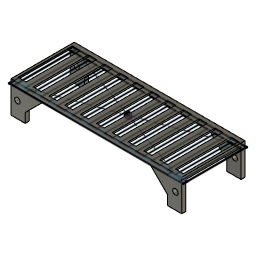
Rear Vent Grill (2mm Smaller) (Autodesk Fusion 360 design; units mm, degrees)
Autodesk Fusion 360 part; units mm, degrees
sketch "Sketch1" plane through (0, 0, 0) normal (0, 0, 1) x (1, 0, 0)
  line L0 (55, -20) -> (-55, -20)
  line L1 (-55, -20) -> (-55, 20)
  line L2 (-55, 20) -> (55, 20)
  line L3 (55, 20) -> (55, -20)
  line L4 (55, -20) -> (-55, 20) construction
  line L5 (-55, -20) -> (55, 20) construction
  line L6 (-55, 20) -> (-52.5, 20)
  line L7 (-52.5, 20) -> (-52.5, -20)
  line L8 (-52.5, -20) -> (-55, -20)
  line L9 (-55, -20) -> (-55, 20)
  line L10 (55, 20) -> (52.5, 20)
  line L11 (52.5, 20) -> (52.5, -20)
  line L12 (52.5, -20) -> (55, -20)
  line L13 (55, -20) -> (55, 20)
  line L14 (-55, 20) -> (55, 20)
  line L15 (55, 20) -> (55, 17.5)
  line L16 (55, 17.5) -> (-55, 17.5)
  line L17 (-55, 17.5) -> (-55, 20)
  line L18 (-55, -20) -> (55, -20)
  line L19 (55, -20) -> (55, -17.5)
  line L20 (55, -17.5) -> (-55, -17.5)
  line L21 (-55, -17.5) -> (-55, -20)
  line L22 (-52.5, 17.5) -> (-47.5, 17.5)
  line L23 (-47.5, 17.5) -> (-47.5, -17.5)
  line L24 (-47.5, -17.5) -> (-52.5, -17.5)
  line L25 (-52.5, -17.5) -> (-52.5, 17.5)
  line L26 (-42.5, -17.5) -> (-42.5, 17.5)
  line L27 (-42.5, 17.5) -> (-37.5, 17.5)
  line L28 (-37.5, 17.5) -> (-37.5, -17.5)
  line L29 (-37.5, -17.5) -> (-42.5, -17.5)
  line L30 (-32.5, -17.5) -> (-32.5, 17.5)
  line L31 (-32.5, 17.5) -> (-27.5, 17.5)
  line L32 (-27.5, 17.5) -> (-27.5, -17.5)
  line L33 (-27.5, -17.5) -> (-32.5, -17.5)
  line L34 (-22.5, -17.5) -> (-22.5, 17.5)
  line L35 (-22.5, 17.5) -> (-17.5, 17.5)
  line L36 (-17.5, 17.5) -> (-17.5, -17.5)
  line L37 (-17.5, -17.5) -> (-22.5, -17.5)
  line L38 (-12.5, -17.5) -> (-12.5, 17.5)
  line L39 (-12.5, 17.5) -> (-7.5, 17.5)
  line L40 (-7.5, 17.5) -> (-7.5, -17.5)
  line L41 (-7.5, -17.5) -> (-12.5, -17.5)
  line L42 (-2.5, -17.5) -> (-2.5, 17.5)
  line L43 (-2.5, 17.5) -> (2.5, 17.5)
  line L44 (2.5, 17.5) -> (2.5, -17.5)
  line L45 (2.5, -17.5) -> (-2.5, -17.5)
  line L46 (7.5, -17.5) -> (7.5, 17.5)
  line L47 (7.5, 17.5) -> (12.5, 17.5)
  line L48 (12.5, 17.5) -> (12.5, -17.5)
  line L49 (12.5, -17.5) -> (7.5, -17.5)
  line L50 (17.5, -17.5) -> (17.5, 17.5)
  line L51 (17.5, 17.5) -> (22.5, 17.5)
  line L52 (22.5, 17.5) -> (22.5, -17.5)
  line L53 (22.5, -17.5) -> (17.5, -17.5)
  line L54 (27.5, -17.5) -> (27.5, 17.5)
  line L55 (27.5, 17.5) -> (32.5, 17.5)
  line L56 (32.5, 17.5) -> (32.5, -17.5)
  line L57 (32.5, -17.5) -> (27.5, -17.5)
  line L58 (37.5, -17.5) -> (37.5, 17.5)
  line L59 (37.5, 17.5) -> (42.5, 17.5)
  line L60 (42.5, 17.5) -> (42.5, -17.5)
  line L61 (42.5, -17.5) -> (37.5, -17.5)
  line L62 (47.5, -17.5) -> (47.5, 17.5)
  line L63 (47.5, 17.5) -> (52.5, 17.5)
  line L64 (52.5, 17.5) -> (52.5, -17.5)
  line L65 (52.5, -17.5) -> (47.5, -17.5)
  line L66 (-55, -20) -> (-45, -20)
  line L67 (-45, -20) -> (-45, -17)
  line L68 (-45, -17) -> (-55, -17)
  line L69 (-55, -17) -> (-55, -20)
  line L70 (-55, 20) -> (-45, 20)
  line L71 (-45, 20) -> (-45, 17)
  line L72 (-45, 17) -> (-55, 17)
  line L73 (-55, 17) -> (-55, 20)
  line L74 (55, -20) -> (45, -20)
  line L75 (45, -20) -> (45, -17)
  line L76 (45, -17) -> (55, -17)
  line L77 (55, -17) -> (55, -20)
  line L78 (55, 20) -> (45, 20)
  line L79 (45, 20) -> (45, 17)
  line L80 (45, 17) -> (55, 17)
  line L81 (55, 17) -> (55, 20)
  dimension "d1" = 40
  dimension "d2" = 110
  dimension "d3" = 2.5
  dimension "d4" = 2.5
  dimension "d5" = 2.5
  dimension "d6" = 2.5
  dimension "d7" = 5
  dimension "d10" = 100
  dimension "d11" = 0
  dimension "d14" = 3
  dimension "d15" = 10
  dimension "d16" = 10
  dimension "d17" = 3
  dimension "d18" = 10
  dimension "d19" = 3
  dimension "d20" = 3
  dimension "d21" = 10
  constraint perpendicular L0 L1
  constraint parallel L0 L2
  constraint parallel L1 L3
  constraint horizontal L0
  constraint coincident L4 origin
  constraint coincident L5 origin
  constraint horizontal L6
  constraint vertical L7
  constraint horizontal L8
  constraint vertical L9
  constraint horizontal L10
  constraint vertical L11
  constraint horizontal L12
  constraint vertical L13
  constraint horizontal L14
  constraint vertical L15
  constraint horizontal L16
  constraint vertical L17
  constraint horizontal L18
  constraint vertical L19
  constraint horizontal L20
  constraint vertical L21
  constraint horizontal L22
  constraint vertical L23
  constraint horizontal L24
  constraint vertical L25
  constraint coincident L7 L22.start
  constraint coincident L16 L22.start
  constraint horizontal L66
  constraint vertical L67
  constraint horizontal L68
  constraint vertical L69
  constraint horizontal L70
  constraint vertical L71
  constraint horizontal L72
  constraint vertical L73
  constraint horizontal L74
  constraint vertical L75
  constraint horizontal L76
  constraint vertical L77
  constraint horizontal L78
  constraint vertical L79
  constraint horizontal L80
  constraint vertical L81
  measures "d1" distance of L0.end L1.end
  measures "d2" distance of L1.end L2.end
  measures "d3" distance of L1.end L6.end
  measures "d4" distance of L2.end L10.end
  measures "d5" distance of L1.end L16.end
  measures "d6" distance of L0.end L20.end
  measures "d7" distance of L22.start L22.end
  measures "d14" distance of L0.end L68.end
  measures "d15" distance of L0.end L66.end
  measures "d16" distance of L1.end L70.end
  measures "d17" distance of L1.end L72.end
  measures "d18" distance of L0.start L74.end
  measures "d19" distance of L0.start L76.end
  measures "d20" distance of L2.end L80.end
  measures "d21" distance of L2.end L78.end
extrude "Extrude1" add sketch "Sketch1" along normal blind 3 contours L0 L3 L11 L12 L13 L18 L19 L20 L74 L77 | L0 L11 L18 L20 L65 L74 L75 | L3 L11 L13 L20 L64 L76 L77 | L0 L18 L20 L29 L33 L37 L41 L45 L49 L53 L57 L61 L67 L75 | L3 L11 L13 L64 L76 L80 | L0 L7 L18 L20 L24 L66 L67 | L20 L62 L75 L76 | L16 L20 L60 L62 L75 L76 L79 L80 | L3 L11 L13 L16 L64 L80 L81 | L0 L1 L7 L8 L9 L18 L20 L21 L66 L69 | L16 L20 L23 L26 L67 L68 L71 L72 | L2 L3 L10 L11 L13 L14 L15 L16 L78 L81 | L1 L7 L9 L20 L25 L68 L69 | L7 L20 L23 L24 L25 L68 | L16 L20 L56 L58 | L2 L14 L16 L27 L31 L35 L39 L43 L47 L51 L55 L59 L71 L79 | L2 L11 L14 L16 L63 L78 L79 | L16 L62 L79 L80 | L1 L7 L9 L25 L68 L72 | L16 L20 L28 L30 | L1 L7 L9 L16 L25 L72 L73 | L7 L16 L22 L23 L25 L72 | L2 L7 L14 L16 L22 L70 L71 | L16 L20 L52 L54 | L1 L2 L6 L7 L9 L14 L16 L17 L70 L73 | L16 L20 L32 L34 | L16 L20 L48 L50 | L16 L20 L36 L38 | L16 L20 L44 L46 | L16 L20 L40 L42
extrude "Extrude2" add sketch "Sketch1" against normal blind 17 contours L0 L3 L11 L12 L13 L18 L19 L20 L74 L77 | L0 L11 L18 L20 L65 L74 L75 | L0 L7 L18 L20 L24 L66 L67 | L0 L1 L7 L8 L9 L18 L20 L21 L66 L69 | L2 L3 L10 L11 L13 L14 L15 L16 L78 L81 | L2 L11 L14 L16 L63 L78 L79 | L2 L7 L14 L16 L22 L70 L71 | L1 L2 L6 L7 L9 L14 L16 L17 L70 L73
sketch "Sketch2" plane through (0, -20, 0) normal (0, -1, 0) x (1, 0, 0)
  line L0 (-45, 0) -> (45, 0)
  line L1 (45, 0) -> (45, -17)
  line L2 (45, -17) -> (55, -17)
  line L3 (55, -17) -> (55, 3)
  line L4 (55, 3) -> (-55, 3)
  line L5 (-55, 3) -> (-55, -17)
  line L6 (-55, -17) -> (-45, -17)
  line L7 (-45, -17) -> (-45, 0)
  circle A0 centre (-50, -7) radius 1.75
  circle A1 centre (50, -7) radius 1.75
  dimension "d24" = 3.5
  dimension "d25" = 3.5
  dimension "d28" = 10
  dimension "d29" = 10
  dimension "d30" = 5
  dimension "d31" = 5
  measures "d24" diameter of A0
  measures "d25" diameter of A1
  measures "d28" distance of L4 A1.centre
  measures "d29" distance of L4 A0.centre
  measures "d30" distance of L5 A0.centre
  measures "d31" distance of L3 A1.centre
extrude "Extrude3" cut sketch "Sketch2" against normal up to surface (40 mm away) contours A0 | A1
extrude "Extrude4" add 1 faces at (-45.8333, 17, 1) along direction (0, 1, 0) blind 0.5
extrude "Extrude5" add 1 faces at (-45.8333, -17, 1) along direction (0, -1, 0) blind 0.5
chamfer "Chamfer1" distance 2 angle 45 19 edges at (47.5, 0, 0) (42.5, 0, 0) (37.5, 0, 0) (32.5, 0, 0) (22.5, 0, 0) (27.5, 0, 0) (17.5, 0, 0) (12.5, 0, 0) (7.5, 0, 0) (2.5, 0, 0) (-2.5, 0, 0) (-7.5, 0, 0) (-12.5, 0, 0) (-17.5, 0, 0) (-22.5, 0, 0) (-27.5, 0, 0) (-32.5, 0, 0) (-37.5, 0, 0) (-42.5, 0, 0)
chamfer "Chamfer2" distance 2 angle 45 1 edges at (-47.5, 0, 0)
chamfer "Chamfer3" distance 2 angle 45 2 edges at (52.5, 0, 0) (-52.5, 0, 0)
chamfer "Chamfer4" distance 11 angle 45 4 edges at (-45, -18.75, 0) (45, -18.75, 0) (45, 18.75, 0) (-45, 18.75, 0)
extrude "Extrude6" cut 1 faces at (55, 5.8333, 2) along direction (-1, 0, 0) blind 1
extrude "Extrude7" cut 1 faces at (-55, -5.8333, 2) along direction (1, 0, 0) blind 1
